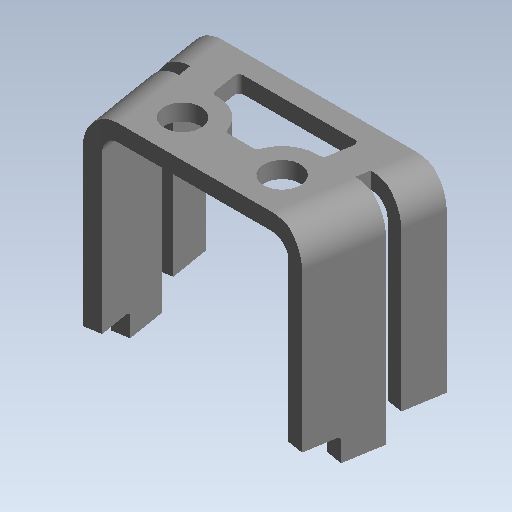
# Autodesk Inventor part: 4463570 DHAS-ME-H9-80---(befestigung)
Saved by Autodesk Inventor 2020 (Build 240168000, 168)
## iProperties
Part Number: 4463570 DHAS-ME-H9-80---(befestigung)
Material: Generic
Catalog Web Link: www.cadenas.de
Description: DHAS-ME_b-mounting kit
Vendor: FESTO
Document SubType Name: Modeling
Designer: partserver
Manufacturer: FESTO
Mass: 1.75982 g
Surface Area: 24.3596 cm^2
Volume: 1.75982 cm^3
Density: 1 g/cm^3
Appearance: PSOLRGB-175-175-175
Category: PARTsolutions
Company: FESTO
PSOL_IDENT_0: {$CADENAS_DATA\23d-libs\festo\parts\d\dhas\parts\dhas_me_befestigung.prj},218 {VTYP=3D},{NB=4463570
PSOL_IDENT_1: DHAS-ME-H9-80---(befestigung)},{LINA=4463570 DHAS-ME-H9-80---(befestigung)},{NN=DHAS-ME_b},{DATE=30.
PSOL_IDENT_2: 08.2019 14:48:26},{GEOMDATE=17.03.2016 08:31:00},{VERSION=},{LINEID=230},{WBVAR=},{WBNUMERIC=}  {NB=
PSOL_IDENT_3: 4463570 DHAS-ME-H9-80---(befestigung)},{LINA=4463570 DHAS-ME-H9-80---(befestigung)},{KT=DUMMY},{TNR=
PSOL_IDENT_4: 4463570},{TYP=DHAS-ME-H9-80},{SIZE=80}
NB: 4463570 DHAS-ME-H9-80---(befestigung)
NN: DHAS-ME_b
NT: mounting kit
NBSYN: $TNR. $TYP.---(befestigung)
LINA: 4463570 DHAS-ME-H9-80---(befestigung)
CATALOG: Festo
TNR: 4463570
TYP: DHAS-ME-H9-80
SIZE: 80
SUPPLIER: FESTO
ARTICLENO: 4463570 DHAS-ME-H9-80---(befestigung)
BOMINFO: 4463570 DHAS-ME-H9-80---(befestigung)
CREATOR: CADENAS GmbH
Title: 4463570 DHAS-ME-H9-80---(befestigung)
Author: Cadenas PARTsolutions
Comments: mounting kit
Autodesk Inventor part; units mm, degrees
ref_plane "YZ Plane" through (0, 0, 0) normal (1, 0, 0) x (0, 1, 0)
ref_plane "XZ Plane" through (0, 0, 0) normal (0, 1, 0) x (-1, 0, 0)
ref_plane "XY Plane" through (0, 0, 0) normal (0, 0, 1) x (1, 0, 0)
sketch "Sketch_1" plane through (0, 0, 0) normal (0, 0, 1) x (1, 0, 0)
  line L0 (11.1731, -15.3) -> (13.2, -15.3)
  line L1 (13.2, -15.3) -> (15.7192, 0)
  line L2 (15.7192, 0) -> (13.6923, 0)
  line L3 (13.6923, 0) -> (11.1731, -15.3)
  constraints: 8 end point
extrude "Extrusion1" add sketch "Sketch_1" along normal blind 25.8
sketch "Sketch_2" plane through (0, 0, 0) normal (0, 0, 1) x (1, 0, 0)
  line L0 (-15.7192, 0) -> (-13.2, -15.3)
  line L1 (-13.2, -15.3) -> (13.2, -15.3)
  line L2 (13.2, -15.3) -> (15.7192, 0)
  line L3 (15.7192, 0) -> (-15.7192, 0)
  constraints: 8 end point
extrude "Extrusion2" add sketch "Sketch_2" along normal blind 2
sketch "Sketch_3" plane through (0, 0, 0) normal (0, 0, 1) x (1, 0, 0)
  line L0 (-15.7192, 0) -> (-13.2, -15.3)
  line L1 (-13.2, -15.3) -> (-11.1731, -15.3)
  line L2 (-11.1731, -15.3) -> (-13.6923, 0)
  line L3 (-13.6923, 0) -> (-15.7192, 0)
  constraints: 8 end point
extrude "Extrusion3" add sketch "Sketch_3" along normal blind 25.8
sketch "Sketch_4" plane through (0, 0, 4) normal (0, 0, 1) x (1, 0, 0)
  line L0 (9.2531, -14.6501) -> (11.7723, 0.6499)
  line L1 (10.8438, -17.3) -> (12.8707, -17.3)
  line L2 (12.8707, -17.3) -> (15.7192, 0)
  line L3 (15.7192, 0) -> (13.6923, 0)
  line L4 (13.6923, 0) -> (10.8438, -17.3)
  constraints: 10 end point
revolve "Revolution1" add sketch "Sketch_4" angle 90 about axis through (9.2531, -14.6501, 4) along (0.162465, 0.9867143, 0)
sketch "Sketch_5" plane through (0, 0, 4) normal (0, 0, 1) x (1, 0, 0)
  line L0 (-11.7723, 0.6499) -> (-9.2531, -14.6501)
  line L1 (-15.7192, 0) -> (-12.8707, -17.3)
  line L2 (-12.8707, -17.3) -> (-10.8438, -17.3)
  line L3 (-10.8438, -17.3) -> (-13.6923, 0)
  line L4 (-13.6923, 0) -> (-15.7192, 0)
  constraints: 10 end point
revolve "Revolution2" add sketch "Sketch_5" angle 90 about axis through (-11.7723, 0.6499, 4) along (0.162465, -0.9867143, 0)
sketch "Sketch_6" plane through (0, 0, 4) normal (0, 0, 1) x (1, 0, 0)
  line L0 (9.2531, -14.6501) -> (11.7723, 0.6499)
  line L1 (12.8707, -17.3) -> (16.9246, -17.3)
  line L2 (16.9246, -17.3) -> (19.773, 0)
  line L3 (19.773, 0) -> (15.7192, 0)
  line L4 (15.7192, 0) -> (12.8707, -17.3)
  constraints: 10 end point
revolve "Revolution3" cut sketch "Sketch_6" angle 90 about axis through (9.2531, -14.6501, 4) along (0.162465, 0.9867143, 0)
sketch "Sketch_7" plane through (0, 0, 4) normal (0, 0, 1) x (1, 0, 0)
  line L0 (-11.7723, 0.6499) -> (-9.2531, -14.6501)
  line L1 (-19.773, 0) -> (-16.9246, -17.3)
  line L2 (-16.9246, -17.3) -> (-12.8707, -17.3)
  line L3 (-12.8707, -17.3) -> (-15.7192, 0)
  line L4 (-15.7192, 0) -> (-19.773, 0)
  constraints: 10 end point
revolve "Revolution4" cut sketch "Sketch_7" angle 90 about axis through (-11.7723, 0.6499, 4) along (0.162465, -0.9867143, 0)
sketch "Sketch_8" plane through (0, 0, 4) normal (0, 0, 1) x (1, 0, 0)
  line L0 (-25, -25) -> (25, -25)
  line L1 (25, -25) -> (25, 5)
  line L2 (25, 5) -> (-25, 5)
  line L3 (-25, 5) -> (-25, -25)
  line L4 (-15.6657, -0.3249) -> (-13.2, -15.3)
  line L5 (-13.2, -15.3) -> (-11.2266, -14.9751)
  line L6 (-11.2266, -14.9751) -> (11.2266, -14.9751)
  line L7 (11.2266, -14.9751) -> (13.2, -15.3)
  line L8 (13.2, -15.3) -> (15.6657, -0.3249)
  line L9 (15.6657, -0.3249) -> (13.6923, 0)
  line L10 (13.6923, 0) -> (-13.6923, 0)
  line L11 (-13.6923, 0) -> (-15.6657, -0.3249)
  constraints: 24 end point
extrude "Extrusion4" cut sketch "Sketch_8" along normal blind 29.8
sketch "Sketch_9" plane through (0, 0, 4) normal (0, 0, 1) x (1, 0, 0)
  line L0 (11.6653, 0) -> (12.4886, 5)
  line L1 (12.4886, 5) -> (16.5424, 5)
  line L2 (16.5424, 5) -> (15.6657, -0.3249)
  line L3 (15.6657, -0.3249) -> (13.6923, 0)
  line L4 (13.6923, 0) -> (11.6653, 0)
  line L5 (11.6653, 0) -> (12.4886, 5)
  constraints: 12 end point
revolve "Revolution5" cut sketch "Sketch_9" angle 360 about axis through (11.6653, 0, 4) along (0.162465, 0.9867143, 0)
sketch "Sketch_10" plane through (0, 0, 4) normal (0, 0, 1) x (1, 0, 0)
  line L0 (-12.4886, 5) -> (-11.6653, 0)
  line L1 (-11.6653, 0) -> (-13.6923, 0)
  line L2 (-13.6923, 0) -> (-15.6657, -0.3249)
  line L3 (-15.6657, -0.3249) -> (-16.5424, 5)
  line L4 (-16.5424, 5) -> (-12.4886, 5)
  line L5 (-12.4886, 5) -> (-11.6653, 0)
  constraints: 12 end point
revolve "Revolution6" cut sketch "Sketch_10" angle 360 about axis through (-12.4886, 5, 4) along (0.162465, -0.9867143, 0)
sketch "Sketch_11" plane through (0, 0, 0) normal (0, 1, 0) x (-1, 0, 0)
  line L0 (30, 6) -> (-30, 6)
  line L1 (-30, 6) -> (-30, -3)
  line L2 (-30, -3) -> (30, -3)
  line L3 (30, -3) -> (30, 6)
  constraints: 8 end point
extrude "Extrusion5" cut sketch "Sketch_11" along normal blind 3
sketch "Sketch_12" plane through (0, 0, 4) normal (0, 0, 1) x (1, 0, 0)
  line L0 (10.6791, -18.3) -> (12.706, -18.3)
  line L1 (12.706, -18.3) -> (13.2, -15.3)
  line L2 (13.2, -15.3) -> (11.2266, -14.9751)
  line L3 (11.2266, -14.9751) -> (10.6791, -18.3)
  constraints: 8 end point
extrude "Extrusion6" cut sketch "Sketch_12" against normal blind 6
sketch "Sketch_13" plane through (0, 0, 4) normal (0, 0, 1) x (1, 0, 0)
  line L0 (-13.2, -15.3) -> (-12.706, -18.3)
  line L1 (-12.706, -18.3) -> (12.706, -18.3)
  line L2 (12.706, -18.3) -> (13.2, -15.3)
  line L3 (13.2, -15.3) -> (11.2266, -14.9751)
  line L4 (11.2266, -14.9751) -> (9.1955, -15)
  line L5 (9.1955, -15) -> (-9.1955, -15)
  line L6 (-9.1955, -15) -> (-11.2266, -14.9751)
  line L7 (-11.2266, -14.9751) -> (-13.2, -15.3)
  constraints: 16 end point
extrude "Extrusion7" cut sketch "Sketch_13" along normal mid plane 12
sketch "Sketch_14" plane through (0, 0, 0) normal (0, 0, 1) x (1, 0, 0)
  line L0 (-25, -25) -> (25, -25)
  line L1 (25, -25) -> (25, 5)
  line L2 (25, 5) -> (-25, 5)
  line L3 (-25, 5) -> (-25, -25)
  line L4 (-15.6657, -0.3249) -> (-14.8918, -5.0249)
  line L5 (-14.8918, -5.0249) -> (-12.9184, -4.7)
  line L6 (-12.9184, -4.7) -> (-10.8915, -4.7)
  line L7 (-10.8915, -4.7) -> (-10.628, -6.3)
  line L8 (-10.628, -6.3) -> (-12.6549, -6.3)
  line L9 (-12.6549, -6.3) -> (-14.6284, -6.6249)
  line L10 (-14.6284, -6.6249) -> (-13.2, -15.3)
  line L11 (-13.2, -15.3) -> (13.2, -15.3)
  line L12 (13.2, -15.3) -> (14.6284, -6.6249)
  line L13 (14.6284, -6.6249) -> (12.6549, -6.3)
  line L14 (12.6549, -6.3) -> (10.628, -6.3)
  line L15 (10.628, -6.3) -> (10.8915, -4.7)
  line L16 (10.8915, -4.7) -> (12.9184, -4.7)
  line L17 (12.9184, -4.7) -> (14.8918, -5.0249)
  line L18 (14.8918, -5.0249) -> (15.6657, -0.3249)
  line L19 (15.6657, -0.3249) -> (13.6923, 0)
  line L20 (13.6923, 0) -> (-13.6923, 0)
  line L21 (-13.6923, 0) -> (-15.6657, -0.3249)
  constraints: 44 end point
extrude "Extrusion8" cut sketch "Sketch_14" along normal blind 29
sketch "Sketch_15" plane through (0, 0, 0) normal (1, 0, 0) x (0, 1, 0)
  line L0 (-27, 33) -> (-27, 23)
  line L1 (-27, 23) -> (-15.5, 23)
  line L2 (-15.5, 23) -> (-15.5, 28)
  line L3 (-15.5, 28) -> (-5.5, 28)
  line L4 (-5.5, 28) -> (-5.5, 23)
  line L5 (-5.5, 23) -> (3, 23)
  line L6 (3, 23) -> (3, 33)
  line L7 (3, 33) -> (-27, 33)
  constraints: 16 end point
extrude "Extrusion9" cut sketch "Sketch_15" along normal mid plane 50
sketch "Sketch16" plane through (0, 0, 0) normal (0, 0, -1) x (-1, 0, 0)
  point P0 (-6, -10.5)
hole "Hole1" at (6, -10.5, 0) direction (0, 0, 1) diameter 4.4 depth 2
sketch "Sketch17" plane through (0, 0, 0) normal (0, 0, -1) x (-1, 0, 0)
  point P0 (6, -10.5)
hole "Hole2" at (-6, -10.5, 0) direction (0, 0, 1) diameter 4.4 depth 2
sketch "Sketch_21" plane through (0, 0, 0) normal (0, 0, 1) x (1, 0, 0)
  arc A0 (-6.7364, -2.45) -> (-7.2298, -3.0312) centre (-6.7364, -2.95) ccw
  line L0 (-7.2298, -3.0312) -> (-6.7687, -5.8312)
  arc A1 (-6.7687, -5.8312) -> (-6.2754, -6.25) centre (-6.2754, -5.75) ccw
  line L1 (-6.2754, -6.25) -> (-6, -6.25)
  arc A2 (-1.9826, -9.1132) -> (-6, -6.25) centre (-6, -10.5) ccw
  arc A3 (-1.9826, -9.1132) -> (-1.51, -9.45) centre (-1.51, -8.95) ccw
  line L2 (-1.51, -9.45) -> (1.51, -9.45)
  arc A4 (1.51, -9.45) -> (1.9826, -9.1132) centre (1.51, -8.95) ccw
  arc A5 (6, -6.25) -> (1.9826, -9.1132) centre (6, -10.5) ccw
  line L3 (6, -6.25) -> (6.2754, -6.25)
  arc A6 (6.2754, -6.25) -> (6.7687, -5.8312) centre (6.2754, -5.75) ccw
  line L4 (6.7687, -5.8312) -> (7.2298, -3.0312)
  arc A7 (7.2298, -3.0312) -> (6.7364, -2.45) centre (6.7364, -2.95) ccw
  line L5 (6.7364, -2.45) -> (-6.7364, -2.45)
  constraints: 16 point on circle, 12 end point, 8 centre point
extrude "Extrusion10" cut sketch "Sketch_21" along normal blind 2
sketch "Sketch_20" plane through (13.2, -15.3, 0) normal (-0.9867143, 0.162465, 0) x (0, 0, -1)
  line L0 (-28, -4.1) -> (-23.5, -4.1)
  arc A0 (-23.5, -4.1) -> (-23, -3.6) centre (-23.5, -3.6) ccw
  line L1 (-23, -3.6) -> (-23, 0)
  line L2 (-23, 0) -> (-28, 0)
  line L3 (-28, 0) -> (-28, -4.1)
  constraints: 8 end point, 2 point on circle, 1 centre point
extrude "Extrusion11" cut sketch "Sketch_20" along normal blind 2
sketch "Sketch_22" plane through (-13.2, -15.3, 0) normal (-0.9867143, -0.162465, 0) x (0, 0, -1)
  line L0 (-28, -4.1) -> (-23.5, -4.1)
  arc A0 (-23.5, -4.1) -> (-23, -3.6) centre (-23.5, -3.6) ccw
  line L1 (-23, -3.6) -> (-23, 0)
  line L2 (-23, 0) -> (-28, 0)
  line L3 (-28, 0) -> (-28, -4.1)
  constraints: 8 end point, 2 point on circle, 1 centre point
extrude "Extrusion12" cut sketch "Sketch_22" against normal blind 2
ref_plane "ANBAU_XY" through (0, -10.5, 0) normal (0, 0, 1) x (1, 0, 0)
ref_plane "ANBAU_YZ" through (0, -10.5, 0) normal (1, 0, 0) x (0, 1, 0)
ref_plane "ANBAU_ZX" through (0, -10.5, 0) normal (0, 1, 0) x (0, 0, 1)
ref_plane "DIN933_1_XY" through (-6, -10.5, 0) normal (0, 0, 1) x (1, 0, 0)
ref_plane "DIN933_1_YZ" through (-6, -10.5, 0) normal (1, 0, 0) x (0, 1, 0)
ref_plane "DIN933_1_ZX" through (-6, -10.5, 0) normal (0, 1, 0) x (0, 0, 1)
ref_plane "DIN933_2_XY" through (6, -10.5, 0) normal (0, 0, 1) x (1, 0, 0)
ref_plane "DIN933_2_YZ" through (6, -10.5, 0) normal (1, 0, 0) x (0, 1, 0)
ref_plane "DIN933_2_ZX" through (6, -10.5, 0) normal (0, 1, 0) x (0, 0, 1)
body "Solid1"
